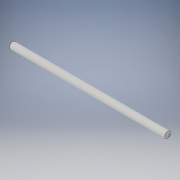
# Autodesk Inventor part: Roller
Saved by Autodesk Inventor 2019.4 (Build 234330000, 330)
## iProperties
Created: 2020-01-11
Part Number: Roller
Material: Generic
Document SubType Name: Modeling
Designer: admin
Density: 1 g/cm^3
Appearance: Default
Author: admin
Autodesk Inventor part; units mm, degrees
ref_plane "YZ Plane" through (0, 0, 0) normal (1, 0, 0) x (0, 1, 0)
ref_plane "XZ Plane" through (0, 0, 0) normal (0, 1, 0) x (-1, 0, 0)
ref_plane "XY Plane" through (0, 0, 0) normal (0, 0, 1) x (1, 0, 0)
sketch "Sketch1" plane through (0, 0, 0) normal (0, 0, 1) x (1, 0, 0)
  line L0 (0, 0) -> (0, 1.4)
  line L1 (0, 1.4) -> (2, 1.4)
  line L2 (2, 1.4) -> (2, 4)
  line L3 (2, 4) -> (195.95, 4)
  line L4 (195.95, 4) -> (195.95, 1.4)
  line L5 (195.95, 1.4) -> (197.45, 1.4)
  line L6 (197.45, 1.4) -> (197.45, 0)
  line L7 (197.45, 0) -> (0, 0)
  dimension "d0" = 1.4
  dimension "d2" = 2
  dimension "d3" = 1.5
  dimension "d4" = 193.95
  dimension "d6" = 4
  constraints: 16 end point, 6 perpendicular, 2 point on line, 1 vertical
  measures "d0" distance of L0.start L0.end
  measures "d2" distance of L0.end L1.end
  measures "d3" distance of L4.end L5.end
  measures "d4" distance between parallel lines of L4 L2
  measures "d6" distance between parallel lines of L7 L3
revolve "Revolution1" add sketch "Sketch1" angle 360 about axis through (197.45, 0, 0) along (-1, 0, 0)
body "Solid1"
